Autodesk Fusion 360 part; units mm, degrees
(part 2 of 2)
sketch "Sketch4" plane through (21.131, -12.2, 0) normal (0.866025, -0.5, 0) x (0.5, 0.866025, 0)
  line L0 (-2.2498, 72.5) -> (-24.0773, 72.5)
  line L1 (-24.0773, 72.5) -> (-24.0773, -1.5)
  line L2 (-24.0773, -1.5) -> (-2.2498, -1.5)
  line L3 (-2.2498, -1.5) -> (-2.2498, 72.5)
  line L4 (-13.1636, -56.7943) -> (-13.1636, 53.7943) construction
  line L5 (-24.0773, 0) -> (-2.2498, 0)
  line L6 (-24.0773, 1.5) -> (-2.2498, 1.5)
  line L7 (-24.0773, 6.3182) -> (-2.2498, 6.3182)
  line L8 (-24.0773, 7.8182) -> (-2.2009, 7.8182)
  line L9 (-29, 10.2273) -> (3, 10.2273) construction
  line L10 (-24.0773, 12.6364) -> (-2.2009, 12.6364)
  line L11 (-24.0773, 14.1364) -> (-2.2498, 14.1364)
  line L12 (-24.0773, 18.9545) -> (-2.2498, 18.9545)
  line L13 (-24.0773, 20.4545) -> (-2.2498, 20.4545)
  line L14 (-24.0773, 22.8636) -> (5, 22.8636) construction
  line L15 (-24.0773, 45.7273) -> (-2.2498, 45.7273)
  line L16 (-24.0773, 44.2273) -> (-2.2498, 44.2273)
  line L17 (-24.0773, 39.4091) -> (-2.2498, 39.4091)
  line L18 (-24.0773, 37.9091) -> (-2.2009, 37.9091)
  line L19 (-24.0773, 33.0909) -> (-2.2009, 33.0909)
  line L20 (-24.0773, 31.5909) -> (-2.2498, 31.5909)
  line L21 (-24.0773, 26.7727) -> (-2.2498, 26.7727)
  line L22 (-24.0773, 25.2727) -> (-2.2498, 25.2727)
  line L23 (-24.0773, 48.1364) -> (-2.2498, 48.1364) construction
  line L24 (-24.0773, 50.5455) -> (-2.2498, 50.5455)
  line L25 (-24.0773, 52.0455) -> (-2.2498, 52.0455)
  line L26 (-24.0773, 56.8636) -> (-2.2498, 56.8636)
  line L27 (-24.0773, 58.3636) -> (-2.2009, 58.3636)
  line L28 (-24.0773, 63.1818) -> (-2.2009, 63.1818)
  line L29 (-24.0773, 64.6818) -> (-2.2498, 64.6818)
  line L30 (-24.0773, 69.5) -> (-2.2498, 69.5)
  line L31 (-21.6894, -1.5) -> (-21.6894, 72.5)
  line L32 (-20.1894, 72.5) -> (-20.1894, -1.5)
  line L33 (-17.8015, -1.5) -> (-17.8015, 72.5)
  line L34 (-17.0515, 74) -> (-17.0515, -4) construction
  line L35 (-16.3015, -1.5) -> (-16.3015, 72.5)
  line L36 (-13.9136, 72.5) -> (-13.9136, -1.5)
  line L37 (-12.4136, -1.5) -> (-12.4136, 72.5)
  line L38 (-10.0257, 72.5) -> (-10.0257, -1.5)
  line L39 (-9.2757, 73) -> (-9.2757, -3.5) construction
  line L40 (-8.5257, 72.5) -> (-8.5257, -1.5)
  line L41 (-6.1378, -1.5) -> (-6.1378, 72.5)
  line L42 (-4.6378, 72.5) -> (-4.6378, -1.5)
  point P0 (-13.1636, -1.5)
  point P1 (-2.2498, 35.5)
  dimension "d35" = 1.5
  dimension "d36" = 1.5
  dimension "d37" = 1.5
  dimension "d38" = 4.8182
  dimension "d39" = 2.4091
  dimension "d40" = 2.4091
  dimension "d42" = 2.4091
  dimension "d44" = 4.8182
  dimension "mezera_svislaa" = 2.3879
  dimension "d48" = 2.3879
  dimension "d49" = 1.5
  dimension "d50" = 0.75
  dimension "d51" = 0.75
  dimension "d99" = 21.8275
  constraint midpoint L2 P0
  constraint midpoint L3 P1
  constraint perpendicular L0 L4
  constraint midpoint P0 L4
  constraint coincident L1 L5.start
  constraint coincident L3 L5.end
  constraint perpendicular L3 L5
  constraint coincident L1 L6.start
  constraint coincident L3 L6.end
  constraint perpendicular L3 L6
  constraint coincident L1 L7.start
  constraint coincident L3 L7.end
  constraint perpendicular L3 L7
  constraint coincident L1 L8.start
  constraint perpendicular L4 L8
  constraint perpendicular L3 L9
  constraint symmetric L5.start L9 L13.start
  constraint symmetric L5.end L9 L13.end
  constraint symmetric L6.start L9 L12.start
  constraint symmetric L6.end L9 L12.end
  constraint symmetric L7.start L9 L11.start
  constraint symmetric L7.end L9 L11.end
  constraint symmetric L8.start L9 L10.start
  constraint symmetric L8.end L9 L10.end
  constraint coincident L1 L14.start
  constraint perpendicular L4 L14
  constraint symmetric L5.start L14 L15.start
  constraint symmetric L5.end L14 L15.end
  constraint symmetric L6.start L14 L16.start
  constraint symmetric L6.end L14 L16.end
  constraint symmetric L7.start L14 L17.start
  constraint symmetric L7.end L14 L17.end
  constraint symmetric L8.start L14 L18.start
  constraint symmetric L8.end L14 L18.end
  constraint symmetric L10.start L14 L19.start
  constraint symmetric L10.end L14 L19.end
  constraint symmetric L11.start L14 L20.start
  constraint symmetric L11.end L14 L20.end
  constraint symmetric L12.start L14 L21.start
  constraint symmetric L12.end L14 L21.end
  constraint symmetric L13.start L14 L22.start
  constraint symmetric L13.end L14 L22.end
  constraint coincident L1 L23.start
  constraint coincident L3 L23.end
  constraint perpendicular L3 L23
  constraint symmetric L15.start L23 L24.start
  constraint symmetric L15.end L23 L24.end
  constraint symmetric L16.start L23 L25.start
  constraint symmetric L16.end L23 L25.end
  constraint symmetric L17.start L23 L26.start
  constraint symmetric L17.end L23 L26.end
  constraint symmetric L18.start L23 L27.start
  constraint symmetric L18.end L23 L27.end
  constraint symmetric L19.start L23 L28.start
  constraint symmetric L19.end L23 L28.end
  constraint symmetric L20.start L23 L29.start
  constraint symmetric L20.end L23 L29.end
  constraint coincident L1 L30.start
  constraint coincident L3 L30.end
  constraint perpendicular L3 L30
  constraint coincident L2 L31.start
  constraint coincident L0 L31.end
  constraint perpendicular L0 L31
  constraint coincident L0 L32.start
  constraint coincident L2 L32.end
  constraint perpendicular L2 L32
  constraint coincident L2 L33.start
  constraint coincident L0 L33.end
  constraint perpendicular L0 L33
  constraint perpendicular L9 L34
  constraint symmetric L0.end L34 L38.start
  constraint symmetric L1.end L34 L38.end
  constraint symmetric L31.start L34 L37.start
  constraint symmetric L31.end L34 L37.end
  constraint symmetric L32.start L34 L36.start
  constraint symmetric L32.end L34 L36.end
  constraint symmetric L33.start L34 L35.start
  constraint symmetric L33.end L34 L35.end
  constraint perpendicular L2 L39
  constraint symmetric L36.start L39 L42.start
  constraint symmetric L36.end L39 L42.end
  constraint symmetric L37.start L39 L41.start
  constraint symmetric L37.end L39 L41.end
  constraint symmetric L38.start L39 L40.start
  constraint symmetric L38.end L39 L40.end
  measures "d35" distance of L5 L6
  measures "d36" distance of L2 L5
  measures "d37" distance of L7 L8
  measures "d38" distance of L6 L7
  measures "d39" distance of L8 L9
  measures "d40" distance of L13 L14
  measures "d42" distance of L15 L23
  measures "d44" distance of L29 L30
  measures "mezera_svislaa" distance of L1 L31
  measures "d48" distance of L32 L33
  measures "d49" distance of L31 L32
  measures "d50" distance of L33 L34
  measures "d51" distance of L38 L39
  measures "d99" distance of L1 L3
extrude "Extrude4" cut sketch "Sketch4" against normal blind 1.5 contours L3 L29 L30 L42 | L29 L30 L40 L41 | L3 L27 L28 L42 | L29 L30 L37 L38 | L27 L28 L40 L41 | L3 L25 L26 L42 | L29 L30 L35 L36 | L27 L28 L37 L38 | L25 L26 L40 L41 | L3 L15 L24 L42 | L29 L30 L32 L33 | L27 L28 L35 L36 | L25 L26 L37 L38 | L15 L24 L40 L41 | L3 L16 L17 L42 | L1 L29 L30 L31 | L27 L28 L32 L33 | L25 L26 L35 L36 | L15 L24 L37 L38 | L16 L17 L40 L41 | L3 L18 L19 L42 | L1 L27 L28 L31 | L25 L26 L32 L33 | L15 L24 L35 L36 | L16 L17 L37 L38 | L18 L19 L40 L41 | L3 L20 L21 L42 | L1 L25 L26 L31 | L15 L24 L32 L33 | L16 L17 L35 L36 | L18 L19 L37 L38 | L20 L21 L40 L41 | L3 L13 L22 L42 | L1 L15 L24 L31 | L16 L17 L32 L33 | L18 L19 L35 L36 | L20 L21 L37 L38 | L13 L22 L40 L41 | L3 L11 L12 L42 | L1 L16 L17 L31 | L18 L19 L32 L33 | L20 L21 L35 L36 | L13 L22 L37 L38 | L11 L12 L40 L41 | L3 L8 L10 L42 | L1 L18 L19 L31 | L20 L21 L32 L33 | L13 L22 L35 L36 | L11 L12 L37 L38 | L8 L10 L40 L41 | L3 L6 L7 L42 | L1 L20 L21 L31 | L13 L22 L32 L33 | L11 L12 L35 L36 | L8 L10 L37 L38 | L6 L7 L40 L41 | L1 L13 L22 L31 | L11 L12 L32 L33 | L8 L10 L35 L36 | L6 L7 L37 L38 | L1 L11 L12 L31 | L8 L10 L32 L33 | L6 L7 L35 L36 | L1 L8 L10 L31 | L6 L7 L32 L33 | L1 L6 L7 L31 bodies 1
sketch "Sketch7" plane through (0, 1.6, 0) normal (0, 1, 0) x (-1, 0, 0)
  line L0 (10.9137, 72.5) -> (-10.9137, 72.5)
  line L1 (-10.9137, 72.5) -> (-10.9137, -1.5)
  line L2 (-10.9137, -1.5) -> (10.9137, -1.5)
  line L3 (10.9137, -1.5) -> (10.9137, 72.5)
  line L4 (-0.75, 80) -> (-0.75, -1.5)
  line L5 (4.6379, 80) -> (4.6379, -1.5)
  line L6 (-10.9137, 56.8636) -> (10.9137, 56.8636)
  line L7 (-10.9137, 63.1818) -> (10.9626, 63.1818)
  line L8 (0.75, -1.5) -> (0.75, 80)
  line L9 (-7.0258, 80) -> (-7.0258, -1.5)
  line L10 (-10.9137, 48.1364) -> (10.9137, 48.1364) construction
  line L11 (-3.8879, 74) -> (-3.8879, -4) construction
  line L12 (-10.9137, 37.9091) -> (10.9626, 37.9091)
  line L13 (-10.9137, 39.4091) -> (10.9137, 39.4091)
  line L14 (3.1379, 80) -> (3.1379, -1.5)
  line L15 (-10.9137, 52.0455) -> (10.9137, 52.0455)
  line L16 (-3.1379, -1.5) -> (-3.1379, 80)
  line L17 (3.8879, 73) -> (3.8879, -3.5) construction
  line L18 (7.0258, -1.5) -> (7.0258, 80)
  line L19 (8.5258, 80) -> (8.5258, -1.5)
  line L20 (-10.9137, 64.6818) -> (10.9137, 64.6818)
  line L21 (-10.9137, 80) -> (-10.9137, -1.5)
  line L22 (-10.9137, 33.0909) -> (10.9626, 33.0909)
  line L23 (-10.9137, 50.5455) -> (10.9137, 50.5455)
  line L24 (-10.9137, -1.5) -> (10.9137, -1.5)
  line L25 (-4.6379, -1.5) -> (-4.6379, 80)
  line L26 (-10.9137, 45.7273) -> (10.9137, 45.7273)
  line L27 (-10.9137, 44.2273) -> (10.9137, 44.2273)
  line L28 (-8.5258, -1.5) -> (-8.5258, 80)
  line L29 (10.9137, -1.5) -> (10.9137, 80)
  line L30 (-15.8364, 10.2273) -> (16.1636, 10.2273) construction
  line L31 (-10.9137, 22.8636) -> (18.1636, 22.8636) construction
  line L32 (-10.9137, 14.1364) -> (10.9137, 14.1364)
  line L33 (-10.9137, 18.9545) -> (10.9137, 18.9545)
  line L34 (-10.9137, 1.5) -> (10.9137, 1.5)
  line L35 (-10.9137, 26.7727) -> (10.9137, 26.7727)
  line L36 (-10.9137, 20.4545) -> (10.9137, 20.4545)
  line L37 (-10.9137, 12.6364) -> (10.9626, 12.6364)
  line L38 (-10.9137, 6.3182) -> (10.9137, 6.3182)
  line L39 (-10.9137, 58.3636) -> (10.9626, 58.3636)
  line L40 (10.9137, 80) -> (-10.9137, 80)
  line L41 (-10.9137, 25.2727) -> (10.9137, 25.2727)
  line L42 (-10.9137, 31.5909) -> (10.9137, 31.5909)
  line L43 (-10.9137, 0) -> (10.9137, 0)
  line L44 (-10.9137, 7.8182) -> (10.9626, 7.8182)
  line L45 (-10.9137, 69.5) -> (10.9137, 69.5)
  point P0 (10.9137, 39.25)
  point P1 (0, -1.5)
  point P2 (0, 53.7943)
  point P3 (13.1636, 0)
  dimension "d84" = 1.5
  dimension "d85" = 1.5
  dimension "d86" = 1.5
  dimension "d87" = 4.8182
  dimension "d88" = 2.4091
  dimension "d89" = 2.4091
  dimension "d90" = 2.4091
  dimension "d91" = 4.8182
  dimension "d92" = 2.3879
  dimension "d93" = 2.3879
  dimension "d94" = 1.5
  dimension "d95" = 0.75
  dimension "d96" = 0.75
  constraint midpoint P1 L24
  constraint midpoint P0 L29
  constraint coincident L43.start L21
  constraint coincident L43.end L29
  constraint perpendicular L29 L43
  constraint coincident L34.start L21
  constraint coincident L34.end L29
  constraint perpendicular L29 L34
  constraint coincident L38.start L21
  constraint coincident L38.end L29
  constraint perpendicular L29 L38
  constraint coincident L44.start L21
  constraint perpendicular L29 L30
  constraint symmetric L43.start L36.start L30
  constraint symmetric L43.end L36.end L30
  constraint symmetric L34.start L33.start L30
  constraint symmetric L34.end L33.end L30
  constraint symmetric L38.start L32.start L30
  constraint symmetric L38.end L32.end L30
  constraint symmetric L44.start L37.start L30
  constraint symmetric L44.end L37.end L30
  constraint coincident L31.start L21
  constraint symmetric L43.start L26.start L31
  constraint symmetric L43.end L26.end L31
  constraint symmetric L34.start L27.start L31
  constraint symmetric L34.end L27.end L31
  constraint symmetric L38.start L13.start L31
  constraint symmetric L38.end L13.end L31
  constraint symmetric L44.start L12.start L31
  constraint symmetric L44.end L12.end L31
  constraint symmetric L22.start L37.start L31
  constraint symmetric L22.end L37.end L31
  constraint symmetric L42.start L32.start L31
  constraint symmetric L42.end L32.end L31
  constraint symmetric L35.start L33.start L31
  constraint symmetric L35.end L33.end L31
  constraint symmetric L36.start L41.start L31
  constraint symmetric L36.end L41.end L31
  constraint coincident L10.start L21
  constraint coincident L10.end L29
  constraint perpendicular L10 L29
  constraint symmetric L23.start L26.start L10
  constraint symmetric L23.end L26.end L10
  constraint symmetric L15.start L27.start L10
  constraint symmetric L15.end L27.end L10
  constraint symmetric L6.start L13.start L10
  constraint symmetric L6.end L13.end L10
  constraint symmetric L39.start L12.start L10
  constraint symmetric L39.end L12.end L10
  constraint symmetric L7.start L22.start L10
  constraint symmetric L7.end L22.end L10
  constraint symmetric L20.start L42.start L10
  constraint symmetric L20.end L42.end L10
  constraint coincident L45.start L21
  constraint coincident L45.end L29
  constraint perpendicular L29 L45
  constraint coincident L28.start L24
  constraint coincident L28.end L40
  constraint perpendicular L28 L40
  constraint coincident L9.start L40
  constraint coincident L9.end L24
  constraint perpendicular L9 L24
  constraint coincident L25.start L24
  constraint coincident L25.end L40
  constraint perpendicular L25 L40
  constraint perpendicular L11 L30
  constraint symmetric L14.start L21.start L11
  constraint symmetric L14.end L1.end L11
  constraint symmetric L28.start L8.start L11
  constraint symmetric L28.end L8.end L11
  constraint symmetric L4.start L9.start L11
  constraint symmetric L4.end L9.end L11
  constraint symmetric L25.start L16.start L11
  constraint symmetric L25.end L16.end L11
  constraint perpendicular L17 L24
  constraint symmetric L19.start L4.start L17
  constraint symmetric L19.end L4.end L17
  constraint symmetric L18.start L8.start L17
  constraint symmetric L18.end L8.end L17
  constraint symmetric L5.start L14.start L17
  constraint symmetric L5.end L14.end L17
  measures "d84" distance of L34 L43
  measures "d85" distance of L24 L43
  measures "d86" distance of L38 L44
  measures "d87" distance of L34 L38
  measures "d88" distance of L30 L44
  measures "d89" distance of L31 L36
  measures "d90" distance of L10 L26
  measures "d91" distance of L20 L45
  measures "d92" distance of L21 L28
  measures "d93" distance of L9 L25
  measures "d94" distance of L9 L28
  measures "d95" distance of L11 L25
  measures "d96" distance of L14 L17
extrude "Extrude7" cut sketch "Sketch7" against normal blind 1.5 contours L3 L19 L20 L29 L45 | L5 L18 L20 L45 | L3 L7 L19 L29 L39 | L8 L14 L20 L45 | L5 L7 L18 L39 | L3 L6 L15 L19 L29 | L4 L16 L20 L45 | L7 L8 L14 L39 | L5 L6 L15 L18 | L3 L19 L23 L26 L29 | L9 L20 L25 L45 | L4 L7 L16 L39 | L6 L8 L14 L15 | L5 L18 L23 L26 | L3 L13 L19 L27 L29 | L1 L20 L21 L28 L45 | L7 L9 L25 L39 | L4 L6 L15 L16 | L8 L14 L23 L26 | L5 L13 L18 L27 | L3 L12 L19 L22 L29 | L1 L7 L21 L28 L39 | L6 L9 L15 L25 | L4 L16 L23 L26 | L8 L13 L14 L27 | L5 L12 L18 L22 | L3 L19 L29 L35 L42 | L1 L6 L15 L21 L28 | L9 L23 L25 L26 | L4 L13 L16 L27 | L8 L12 L14 L22 | L5 L18 L35 L42 | L3 L19 L29 L36 L41 | L1 L21 L23 L26 L28 | L9 L13 L25 L27 | L4 L12 L16 L22 | L8 L14 L35 L42 | L5 L18 L36 L41 | L3 L19 L29 L32 L33 | L1 L13 L21 L27 L28 | L9 L12 L22 L25 | L4 L16 L35 L42 | L8 L14 L36 L41 | L5 L18 L32 L33 | L3 L19 L29 L37 L44 | L1 L12 L21 L22 L28 | L9 L25 L35 L42 | L4 L16 L36 L41 | L8 L14 L32 L33 | L5 L18 L37 L44 | L3 L19 L29 L34 L38 | L1 L21 L28 L35 L42 | L9 L25 L36 L41 | L4 L16 L32 L33 | L8 L14 L37 L44 | L5 L18 L34 L38 | L1 L21 L28 L36 L41 | L9 L25 L32 L33 | L4 L16 L37 L44 | L8 L14 L34 L38 | L1 L21 L28 L32 L33 | L9 L25 L37 L44 | L4 L16 L34 L38 | L1 L21 L28 L37 L44 | L9 L25 L34 L38 | L1 L21 L28 L34 L38 bodies 1
sketch "Sketch8" plane through (-21.131, -12.2, 0) normal (-0.866025, -0.5, 0) x (0.5, -0.866025, 0)
  line L0 (24.0773, 72.5) -> (2.2498, 72.5)
  line L1 (2.2498, 72.5) -> (2.2498, -1.5)
  line L2 (2.2498, -1.5) -> (24.0773, -1.5)
  line L3 (24.0773, -1.5) -> (24.0773, 72.5)
  line L4 (9.2757, 74) -> (9.2757, -4) construction
  line L5 (13.9136, -1.5) -> (13.9136, 80)
  line L6 (2.2498, 45.7273) -> (24.0773, 45.7273)
  line L7 (2.2498, 64.6818) -> (24.0773, 64.6818)
  line L8 (21.6894, 80) -> (21.6894, -1.5)
  line L9 (2.2498, 58.3636) -> (24.1262, 58.3636)
  line L10 (2.2498, 63.1818) -> (24.1262, 63.1818)
  line L11 (6.1378, 80) -> (6.1378, -1.5)
  line L12 (17.8015, 80) -> (17.8015, -1.5)
  line L13 (10.0257, -1.5) -> (10.0257, 80)
  line L14 (2.2498, 52.0455) -> (24.0773, 52.0455)
  line L15 (20.1894, -1.5) -> (20.1894, 80)
  line L16 (2.2498, 48.1364) -> (24.0773, 48.1364) construction
  line L17 (2.2498, 56.8636) -> (24.0773, 56.8636)
  line L18 (2.2498, 50.5455) -> (24.0773, 50.5455)
  line L19 (4.6378, -1.5) -> (4.6378, 80)
  line L20 (2.2498, -1.5) -> (24.0773, -1.5)
  line L21 (2.2498, 69.5) -> (24.0773, 69.5)
  line L22 (24.0773, 80) -> (2.2498, 80)
  line L23 (17.0515, 73) -> (17.0515, -3.5) construction
  line L24 (2.2498, 39.4091) -> (24.0773, 39.4091)
  line L25 (2.2498, 44.2273) -> (24.0773, 44.2273)
  line L26 (24.0773, -1.5) -> (24.0773, 80)
  line L27 (2.2498, 37.9091) -> (24.1262, 37.9091)
  line L28 (16.3015, 80) -> (16.3015, -1.5)
  line L29 (2.2498, 12.6364) -> (24.1262, 12.6364)
  line L30 (8.5257, -1.5) -> (8.5257, 80)
  line L31 (-2.6728, 10.2273) -> (29.3272, 10.2273) construction
  line L32 (2.2498, 80) -> (2.2498, -1.5)
  line L33 (2.2498, 1.5) -> (24.0773, 1.5)
  line L34 (2.2498, 14.1364) -> (24.0773, 14.1364)
  line L35 (12.4136, 80) -> (12.4136, -1.5)
  line L36 (2.2498, 22.8636) -> (31.3272, 22.8636) construction
  line L37 (2.2498, 20.4545) -> (24.0773, 20.4545)
  line L38 (2.2498, 0) -> (24.0773, 0)
  line L39 (2.2498, 31.5909) -> (24.0773, 31.5909)
  line L40 (2.2498, 7.8182) -> (24.1262, 7.8182)
  line L41 (2.2498, 25.2727) -> (24.0773, 25.2727)
  line L42 (2.2498, 33.0909) -> (24.1262, 33.0909)
  line L43 (2.2498, 26.7727) -> (24.0773, 26.7727)
  line L44 (2.2498, 6.3182) -> (24.0773, 6.3182)
  line L45 (2.2498, 18.9545) -> (24.0773, 18.9545)
  point P0 (24.0773, 39.25)
  point P1 (13.1636, -1.5)
  point P2 (13.1636, 53.7943)
  point P3 (26.3272, 0)
  dimension "d100" = 1.5
  dimension "d101" = 1.5
  dimension "d102" = 1.5
  dimension "d103" = 4.8182
  dimension "d104" = 2.4091
  dimension "d105" = 2.4091
  dimension "d106" = 2.4091
  dimension "d107" = 4.8182
  dimension "d108" = 2.3879
  dimension "d109" = 2.3879
  dimension "d110" = 1.5
  dimension "d111" = 0.75
  dimension "d112" = 0.75
  dimension "d113" = 21.8275
  constraint midpoint P1 L20
  constraint midpoint P0 L26
  constraint coincident L38.start L32
  constraint coincident L38.end L26
  constraint perpendicular L26 L38
  constraint coincident L33.start L32
  constraint coincident L33.end L26
  constraint perpendicular L26 L33
  constraint coincident L44.start L32
  constraint coincident L44.end L26
  constraint perpendicular L26 L44
  constraint coincident L40.start L32
  constraint perpendicular L26 L31
  constraint symmetric L38.start L37.start L31
  constraint symmetric L38.end L37.end L31
  constraint symmetric L33.start L45.start L31
  constraint symmetric L33.end L45.end L31
  constraint symmetric L44.start L34.start L31
  constraint symmetric L44.end L34.end L31
  constraint symmetric L40.start L29.start L31
  constraint symmetric L40.end L29.end L31
  constraint coincident L36.start L32
  constraint symmetric L38.start L6.start L36
  constraint symmetric L38.end L6.end L36
  constraint symmetric L33.start L25.start L36
  constraint symmetric L33.end L25.end L36
  constraint symmetric L44.start L24.start L36
  constraint symmetric L44.end L24.end L36
  constraint symmetric L40.start L27.start L36
  constraint symmetric L40.end L27.end L36
  constraint symmetric L42.start L29.start L36
  constraint symmetric L42.end L29.end L36
  constraint symmetric L39.start L34.start L36
  constraint symmetric L39.end L34.end L36
  constraint symmetric L43.start L45.start L36
  constraint symmetric L43.end L45.end L36
  constraint symmetric L37.start L41.start L36
  constraint symmetric L37.end L41.end L36
  constraint coincident L16.start L32
  constraint coincident L16.end L26
  constraint perpendicular L16 L26
  constraint symmetric L18.start L6.start L16
  constraint symmetric L18.end L6.end L16
  constraint symmetric L14.start L25.start L16
  constraint symmetric L14.end L25.end L16
  constraint symmetric L17.start L24.start L16
  constraint symmetric L17.end L24.end L16
  constraint symmetric L9.start L27.start L16
  constraint symmetric L9.end L27.end L16
  constraint symmetric L10.start L42.start L16
  constraint symmetric L10.end L42.end L16
  constraint symmetric L7.start L39.start L16
  constraint symmetric L7.end L39.end L16
  constraint coincident L21.start L32
  constraint coincident L21.end L26
  constraint perpendicular L21 L26
  constraint coincident L19.start L20
  constraint coincident L19.end L22
  constraint perpendicular L19 L22
  constraint coincident L11.start L22
  constraint coincident L11.end L20
  constraint perpendicular L11 L20
  constraint coincident L30.start L20
  constraint coincident L30.end L22
  constraint perpendicular L22 L30
  constraint perpendicular L4 L31
  constraint symmetric L28.start L22.end L4
  constraint symmetric L28.end L1.end L4
  constraint symmetric L19.start L5.start L4
  constraint symmetric L19.end L5.end L4
  constraint symmetric L35.start L11.start L4
  constraint symmetric L35.end L11.end L4
  constraint symmetric L30.start L13.start L4
  constraint symmetric L30.end L13.end L4
  constraint perpendicular L20 L23
  constraint symmetric L8.start L35.start L23
  constraint symmetric L8.end L35.end L23
  constraint symmetric L15.start L5.start L23
  constraint symmetric L15.end L5.end L23
  constraint symmetric L12.start L28.start L23
  constraint symmetric L12.end L28.end L23
  measures "d100" distance of L33 L38
  measures "d101" distance of L20 L38
  measures "d102" distance of L40 L44
  measures "d103" distance of L33 L44
  measures "d104" distance of L31 L40
  measures "d105" distance of L36 L37
  measures "d106" distance of L6 L16
  measures "d107" distance of L7 L21
  measures "d108" distance of L19 L32
  measures "d109" distance of L11 L30
  measures "d110" distance of L11 L19
  measures "d111" distance of L4 L30
  measures "d112" distance of L23 L28
  measures "d113" distance of L26 L32
extrude "Extrude8" cut sketch "Sketch8" against normal blind 1.5 contours L3 L7 L8 L21 L26 | L7 L12 L15 L21 | L3 L8 L9 L10 L26 | L5 L7 L21 L28 | L9 L10 L12 L15 | L3 L8 L14 L17 L26 | L7 L13 L21 L35 | L5 L9 L10 L28 | L12 L14 L15 L17 | L3 L6 L8 L18 L26 | L7 L11 L21 L30 | L9 L10 L13 L35 | L5 L14 L17 L28 | L6 L12 L15 L18 | L3 L8 L24 L25 L26 | L1 L7 L19 L21 L32 | L9 L10 L11 L30 | L13 L14 L17 L35 | L5 L6 L18 L28 | L12 L15 L24 L25 | L3 L8 L26 L27 L42 | L1 L9 L10 L19 L32 | L11 L14 L17 L30 | L6 L13 L18 L35 | L5 L24 L25 L28 | L12 L15 L27 L42 | L3 L8 L26 L39 L43 | L1 L14 L17 L19 L32 | L6 L11 L18 L30 | L13 L24 L25 L35 | L5 L27 L28 L42 | L12 L15 L39 L43 | L3 L8 L26 L37 L41 | L1 L6 L18 L19 L32 | L11 L24 L25 L30 | L13 L27 L35 L42 | L5 L28 L39 L43 | L12 L15 L37 L41 | L3 L8 L26 L34 L45 | L1 L19 L24 L25 L32 | L11 L27 L30 L42 | L13 L35 L39 L43 | L5 L28 L37 L41 | L12 L15 L34 L45 | L3 L8 L26 L29 L40 | L1 L19 L27 L32 L42 | L11 L30 L39 L43 | L13 L35 L37 L41 | L5 L28 L34 L45 | L12 L15 L29 L40 | L3 L8 L26 L33 L44 | L1 L19 L32 L39 L43 | L11 L30 L37 L41 | L13 L34 L35 L45 | L5 L28 L29 L40 | L12 L15 L33 L44 | L1 L19 L32 L37 L41 | L11 L30 L34 L45 | L13 L29 L35 L40 | L5 L28 L33 L44 | L1 L19 L32 L34 L45 | L11 L29 L30 L40 | L13 L33 L35 L44 | L1 L19 L29 L32 L40 | L11 L30 L33 L44 | L1 L19 L32 L33 L44 bodies 1
sketch "Sketch9" plane through (0, 0, 72.5) normal (0, 0, 1) x (-1, 0, 0)
  line L0 (10.7606, -0.1) -> (-10.7606, -0.1)
  arc A0 (-18.6305, 13.5311) -> (-10.7606, -0.1) centre (-8.5459, 10.266) ccw
  line L1 (-18.6305, 13.5311) -> (-7.8699, 32.1689)
  arc A1 (7.8699, 32.1689) -> (-7.8699, 32.1689) centre (0, 25.0679) ccw
  line L2 (7.8699, 32.1689) -> (18.6305, 13.5311)
  arc A2 (10.7606, -0.1) -> (18.6305, 13.5311) centre (8.5459, 10.266) ccw
  arc A3 (-20.0061, 14.1484) -> (-10.9137, -1.6) centre (-8.5459, 10.266) ccw
  line L3 (-10.9137, -1.6) -> (10.9137, -1.6)
  arc A4 (10.9137, -1.6) -> (20.0061, 14.1484) centre (8.5459, 10.266) ccw
  line L4 (20.0061, 14.1484) -> (9.0924, 33.0516)
  arc A5 (9.0924, 33.0516) -> (-9.0924, 33.0516) centre (0, 25.0679) ccw
  line L5 (-9.0924, 33.0516) -> (-20.0061, 14.1484)
  line L6 (0, -1.6) -> (0, -15) construction
  line L7 (0, -15) -> (0, 60) construction
  line L8 (14.5492, 23.6) -> (40.2725, 38.4514) construction
  line L9 (40.2725, 38.4514) -> (-33.8465, -4.3413) construction
  line L10 (-14.5492, 23.6) -> (-27.559, 31.1112) construction
  line L11 (-27.559, 31.1112) -> (32.4312, -3.5242) construction
  circle A6 centre (0, -1.6) radius 6.5 construction
  circle A7 centre (0, -5.6) radius 1.25
  line L12 (5, -1.6) -> (5, -5.7533)
  line L13 (0, -8.1) -> (2.5, -7.6)
  line L14 (5, -5.7533) -> (2.5, -7.6)
  line L15 (0, -8.1) -> (-2.5, -7.6)
  line L16 (-5, -5.7533) -> (-2.5, -7.6)
  line L17 (-5, -1.6) -> (-5, -5.7533)
  line L18 (17.0492, 19.2699) -> (20.6461, 21.3465)
  line L19 (20.6461, 21.3465) -> (20.9954, 24.4349)
  line L20 (20.1784, 26.85) -> (20.9954, 24.4349)
  line L21 (20.1784, 26.85) -> (18.4954, 28.7651)
  line L22 (15.6461, 30.0068) -> (18.4954, 28.7651)
  line L23 (12.0492, 27.9301) -> (15.6461, 30.0068)
  circle A8 centre (18.0133, 25.6) radius 1.25
  line L24 (-12.0492, 27.9301) -> (-15.6461, 30.0068)
  line L25 (-15.6461, 30.0068) -> (-18.4954, 28.7651)
  line L26 (-20.1784, 26.85) -> (-18.4954, 28.7651)
  line L27 (-20.1784, 26.85) -> (-20.9954, 24.4349)
  line L28 (-20.6461, 21.3465) -> (-20.9954, 24.4349)
  line L29 (-17.0492, 19.2699) -> (-20.6461, 21.3465)
  circle A9 centre (-18.0133, 25.6) radius 1.25
  point P0 (0, 15.2)
  dimension "d116" = 13
  dimension "d117" = 2.5
  dimension "d119" = 4
  dimension "d120" = 5
  dimension "d121" = 2.5
  dimension "d123" = 360
  constraint midpoint L3 L6.start
  constraint perpendicular L3 L6
  constraint perpendicular L0 L7
  constraint midpoint L4 L8.start
  constraint perpendicular L4 L8
  constraint parallel L8 L9
  constraint midpoint L5 L10.start
  constraint perpendicular L5 L10
  constraint parallel L10 L11
  constraint coincident L7 P0
  constraint coincident L11 P0
  constraint coincident L6.start A6.centre
  constraint coincident L7 A7.centre
  constraint coincident L3 L12.start
  constraint coincident A6 L12.end
  constraint perpendicular L3 L12
  constraint coincident A6 L13.start
  constraint coincident L7 L13.start
  constraint coincident A6 L13.end
  constraint symmetric L6 L12.start L17.start
  constraint symmetric L6 L12.end L16.start
  constraint symmetric L6 L13.start L15.start
  constraint symmetric L6 L13.end L15.end
  measures "d116" diameter of A6
  measures "d117" diameter of A7
  measures "d119" distance of L3 A7.centre
  measures "d120" distance of L6 L12
  measures "d121" distance of L6 L13.end
extrude "Extrude9" add sketch "Sketch9" against normal blind 2 contours L5 L24 L25 L26 L27 L28 L29 | L3 L12 L13 L14 L15 L16 L17 | L4 L18 L19 L20 L21 L22 L23 bodies 1
sketch "Sketch10" plane through (0, 0, 72.5) normal (0, 0, 1) x (1, 0, 0)
  arc A0 (20.0061, -14.1484) -> (10.9137, 1.6) centre (8.5459, -10.266) ccw
  line L0 (20.0061, -14.1484) -> (9.0924, -33.0516)
  arc A1 (-9.0924, -33.0516) -> (9.0924, -33.0516) centre (0, -25.0679) ccw
  line L1 (-9.0924, -33.0516) -> (-20.0061, -14.1484)
  arc A2 (-10.9137, 1.6) -> (-20.0061, -14.1484) centre (-8.5459, -10.266) ccw
  line L2 (-10.9137, 1.6) -> (10.9137, 1.6)
  line L3 (14.5492, -23.6) -> (-26.3572, 0.0173) construction
  line L4 (0, 1.6) -> (0, -40) construction
  line L5 (10, 5.85) -> (-10, 5.85) construction
  line L6 (-10, 5.85) -> (-10, -38.85) construction
  line L7 (-10, -38.85) -> (10, -38.85) construction
  line L8 (10, -38.85) -> (10, 5.85) construction
  line L9 (10, 5.85) -> (-10, -38.85) construction
  line L10 (-10, 5.85) -> (10, -38.85) construction
  line L11 (-11, -39.85) -> (11, -39.85)
  line L12 (11, -39.85) -> (11, 6.85)
  line L13 (11, 6.85) -> (-11, 6.85)
  line L14 (-11, 6.85) -> (-11, -39.85)
  circle A3 centre (8.5, 4.35) radius 1.025
  circle A4 centre (-8.5, 4.35) radius 1.025
  line L15 (0, -16.5) -> (25, -16.5) construction
  circle A5 centre (-8.5, -37.35) radius 1.025
  circle A6 centre (8.5, -37.35) radius 1.025
  point P0 (0, -16.5)
  dimension "d126" = 44.7
  dimension "d127" = 20
  dimension "d128" = 1
  dimension "d129" = 1.5
  dimension "d130" = 1.5
  dimension "d131" = 2.05
  dimension "d135" = 18.1
  constraint midpoint L0 L3.start
  constraint perpendicular L0 L3
  constraint midpoint L2 L4.start
  constraint perpendicular L2 L4
  constraint horizontal L5
  constraint perpendicular L5 L6
  constraint parallel L5 L7
  constraint parallel L6 L8
  constraint coincident L9 P0
  constraint coincident L10 P0
  constraint coincident L4 P0
  constraint symmetric L4 A3 A4
  constraint coincident P0 L15.start
  constraint perpendicular L12 L15
  constraint symmetric A3 L15 A6
  constraint symmetric A4 L15 A5
  measures "d126" distance of L5 L7
  measures "d127" distance of L6 L8
  measures "d129" distance of L5 A3.centre
  measures "d130" distance of L8 A3.centre
  measures "d131" diameter of A3
  measures "d135" distance of L2 L15
extrude "Extrude10" add sketch "Sketch10" along normal blind 1.5 from surface at -74 contours A0 L0 A1 L1 A2 L2 L12 L14 | A0 A2 L2 L12 L13 L14 | L0 A1 L1 L11 L12 L14 bodies 1
sketch "Sketch11" plane through (0, 0, 72.5) normal (0, 0, 1) x (-1, 0, 0)
  circle A0 centre (18.0133, 25.6) radius 1.25
  circle A1 centre (0, -5.6) radius 1.25
  circle A2 centre (-18.0133, 25.6) radius 1.25
  line L0 (10.7606, -0.1) -> (-10.7606, -0.1)
  arc A3 (-18.6305, 13.5311) -> (-10.7606, -0.1) centre (-8.5459, 10.266) ccw
  line L1 (-18.6305, 13.5311) -> (-7.8699, 32.1689)
  arc A4 (7.8699, 32.1689) -> (-7.8699, 32.1689) centre (0, 25.0679) ccw
  line L2 (7.8699, 32.1689) -> (18.6305, 13.5311)
  arc A5 (10.7606, -0.1) -> (18.6305, 13.5311) centre (8.5459, 10.266) ccw
  arc A6 (-20.0061, 14.1484) -> (-10.9137, -1.6) centre (-8.5459, 10.266) ccw
  line L3 (-10.9137, -1.6) -> (-5, -1.6)
  line L4 (-5, -1.6) -> (-5, -5.7533)
  line L5 (-5, -5.7533) -> (-2.5, -7.6)
  line L6 (-2.5, -7.6) -> (0, -8.1)
  line L7 (0, -8.1) -> (2.5, -7.6)
  line L8 (2.5, -7.6) -> (5, -5.7533)
  line L9 (5, -5.7533) -> (5, -1.6)
  line L10 (5, -1.6) -> (10.9137, -1.6)
  arc A7 (10.9137, -1.6) -> (20.0061, 14.1484) centre (8.5459, 10.266) ccw
  line L11 (20.0061, 14.1484) -> (17.0492, 19.2699)
  line L12 (17.0492, 19.2699) -> (20.6461, 21.3465)
  line L13 (20.6461, 21.3465) -> (20.9954, 24.4349)
  line L14 (20.9954, 24.4349) -> (20.1784, 26.85)
  line L15 (20.1784, 26.85) -> (18.4954, 28.7651)
  line L16 (18.4954, 28.7651) -> (15.6461, 30.0068)
  line L17 (15.6461, 30.0068) -> (12.0492, 27.9301)
  line L18 (12.0492, 27.9301) -> (9.0924, 33.0516)
  arc A8 (9.0924, 33.0516) -> (-9.0924, 33.0516) centre (0, 25.0679) ccw
  line L19 (-9.0924, 33.0516) -> (-12.0492, 27.9301)
  line L20 (-12.0492, 27.9301) -> (-15.6461, 30.0068)
  line L21 (-15.6461, 30.0068) -> (-18.4954, 28.7651)
  line L22 (-18.4954, 28.7651) -> (-20.1784, 26.85)
  line L23 (-20.1784, 26.85) -> (-20.9954, 24.4349)
  line L24 (-20.9954, 24.4349) -> (-20.6461, 21.3465)
  line L25 (-20.6461, 21.3465) -> (-17.0492, 19.2699)
  line L26 (-17.0492, 19.2699) -> (-20.0061, 14.1484)
extrude "Extrude1" add sketch "Sketch11" along normal blind 1 separate body makes body 2 in component "Component"
component "Component" placed x (1, 0, 0) y (0, 1, 0) z (0, 0, 1) at (0, 0, 0)
equation "d9 = delka_ploska"
equation "d10 = centre"
equation "d12 = d9"
equation "d13 = d10"
equation "d15 = d9"
equation "d16 = d10"
equation "d18 = polomer * 2"
equation "d19 = d18 / 2"
equation "d22 = vyska"
equation "d24 = okraj"
equation "d26 = -vyska"
equation "centre = 15.2 mm"
equation "polomer = 10.5 mm"
equation "vyska = 72.5 mm"
equation "pricka_tlostka = 1.5 mm"
equation "okraj = 1.5 mm"
equation "d35 = pricka_tlostka"
equation "d36 = okraj"
equation "d37 = pricka_tlostka"
equation "d38 = mezera_mezi_prickami"
equation "d39 = d38 / 2"
equation "d40 = d38 / 2"
equation "mezera_mezi_prickami = ( vyska - ( 2 * pricka_tlostka + okraj ) - 10 * pricka_tlostka ) / 11"
equation "d42 = d38 / 2"
equation "d44 = mezera_mezi_prickami"
equation "mezera_svislaa = ( d99 - 5 * pricka_tlostka ) / 6"
equation "delka_ploska = 21.5 mm"
equation "mezera_svisla = ( delka_ploska - 5 * pricka_tlostka ) / 6"
equation "d48 = mezera_svislaa"
equation "d49 = pricka_tlostka"
equation "d50 = pricka_tlostka / 2"
equation "d51 = pricka_tlostka / 2"
equation "d52 = -okraj"
equation "d84 = pricka_tlostka"
equation "d85 = okraj"
equation "d86 = pricka_tlostka"
equation "d87 = mezera_mezi_prickami"
equation "d88 = d38 / 2"
equation "d89 = d38 / 2"
equation "d90 = d38 / 2"
equation "d91 = mezera_mezi_prickami"
equation "d92 = mezera_svislaa"
equation "d93 = mezera_svislaa"
equation "d94 = pricka_tlostka"
equation "d95 = pricka_tlostka / 2"
equation "d96 = pricka_tlostka / 2"
equation "d100 = pricka_tlostka"
equation "d101 = okraj"
equation "d102 = pricka_tlostka"
equation "d103 = mezera_mezi_prickami"
equation "d104 = d38 / 2"
equation "d105 = d38 / 2"
equation "d106 = d38 / 2"
equation "d107 = mezera_mezi_prickami"
equation "d108 = ( d99 - 5 * pricka_tlostka ) / 6"
equation "d109 = mezera_svislaa"
equation "d110 = pricka_tlostka"
equation "d111 = pricka_tlostka / 2"
equation "d112 = pricka_tlostka / 2"
equation "d114 = -okraj"
equation "d117 = uchycujici_dira"
equation "uchycujici_dira = 2.5 mm"
equation "d121 = d120 / 2"
equation "d132 = -vyska - okraj"
equation "d133 = okraj"
